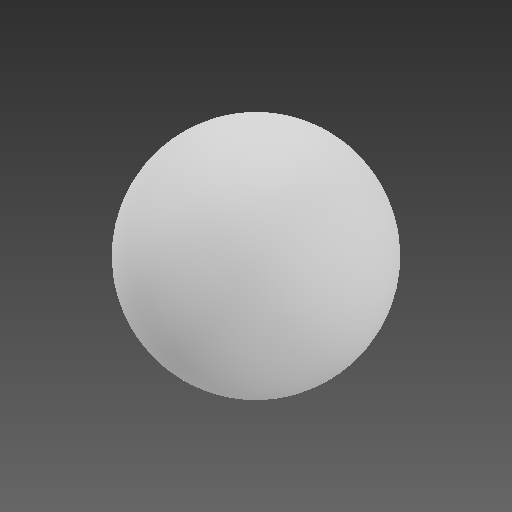
# Autodesk Inventor part: steelBall
Saved by Autodesk Inventor 2021 (Build 250183000, 183)
## iProperties
Created: 2024-03-17
Part Number: steelBall
Material: Generic
Document SubType Name: Modeling
Designer: top10
Density: 1 g/cm^3
Appearance: Default
Author: top10
Autodesk Inventor part; units mm, degrees
ref_plane "YZ Plane" through (0, 0, 0) normal (1, 0, 0) x (0, 1, 0)
ref_plane "XZ Plane" through (0, 0, 0) normal (0, 1, 0) x (-1, 0, 0)
ref_plane "XY Plane" through (0, 0, 0) normal (0, 0, 1) x (1, 0, 0)
sketch "Sketch1" plane through (0, 0, 0) normal (0, 1, 0) x (-1, 0, 0)
  circle A0 centre (0, 0) radius 3.75
  line L0 (0, 9.8946) -> (0, -9.8946)
  point P0 (0, -3.75)
  point P1 (0, 3.75)
  dimension "d0" = 7.5
  constraints: 2 coincident, 2 end point, 2 vertical, 1 centre point, 1 midpoint
  measures "d0" diameter of A0
revolve "Revolution1" add sketch "Sketch1" angle 360 about axis through (0, 0, 9.8946) along (0, 0, -1) picked at (-1.4098, 1.0788) contours L0 A0
body "Solid1"
